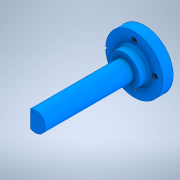
# Autodesk Inventor part: BM-AX12
Saved by Autodesk Inventor 2021 (Build 250183000, 183)
## iProperties
Created: 2021-10-29
Part Number: BM-AX12
Material: PETG
Document SubType Name: Modeling
Designer: Alcatraz
Density: 1.27 g/cm^3
Appearance: Genérico
Author: Alcatraz
Autodesk Inventor part; units mm, degrees
ref_plane "XZ Plane" through (0, 0, 0) normal (0, 1, 0) x (-1, 0, 0)
ref_plane "XY Plane" through (0, 0, 0) normal (0, 0, 1) x (1, 0, 0)
sketch "Boceto1" plane through (0, 0, 0) normal (0, 0, 1) x (1, 0, 0)
  circle A0 centre (0, 0) radius 11
  dimension "DIAMETROBRIDA" = 22
  constraints: 1 centre point, 1 coincident
  measures "DIAMETROBRIDA" diameter of A0
extrude "Extrusión1" add sketch "Boceto1" along normal blind 4
sketch "Boceto2" plane through (0, 0, 4) normal (0, 0, 1) x (1, 0, 0)
  circle A0 centre (0, 8) radius 1.05
  circle A1 centre (-8, 0) radius 1.05
  circle A2 centre (8, 0) radius 1.05
  circle A3 centre (0, -8) radius 1.05
  circle A4 centre (0, 0) radius 11 projected
  dimension "d7" = 2.1
  dimension "d8" = 2.1
  dimension "d9" = 2.1
  dimension "d10" = 2.1
  dimension "DistanciaBarrenos" = 8
  dimension "d31" = 8
  dimension "d32" = 8
  dimension "d33" = 8
  constraints: 4 centre point
  measures "d7" diameter of A0
  measures "d8" diameter of A1
  measures "d9" diameter of A2
  measures "d10" diameter of A3
  measures "DistanciaBarrenos" distance of A1.centre A4.centre
  measures "d31" distance of point (0, 0) A0.centre
  measures "d32" distance of A2.centre point (0, 0)
  measures "d33" distance of A3.centre point (0, 0)
hole "Agujero1" at (0, 8, 4) at (-8, 0, 4) at (8, 0, 4) at (0, -8, 4) direction (0, 0, -1) diameter 2.013 end through all thread size "M2.5x0.45" class "6H" standard "ISO Metric profile"
sketch "Boceto3" plane through (0, 0, 4) normal (0, 0, 1) x (1, 0, 0)
  circle A0 centre (0, 0) radius 6
  dimension "DIAMETROBASE" = 12
  constraints: 1 centre point, 1 coincident
  measures "DIAMETROBASE" diameter of A0
extrude "Extrusión2" add sketch "Boceto3" along normal blind 4
sketch "Boceto4" plane through (0, 0, 8) normal (0, 0, 1) x (1, 0, 0)
  arc A0 (-1.9, -3.2909) -> (-1.9, 3.2909) centre (0, 0) ccw
  line L0 (0, 0) -> (-2, 0)
  line L1 (-1.9, 3.2909) -> (-1.9, -3.2909)
  circle A1 centre (0, 0) radius 6 projected
  dimension "DIAMETROEJE" = 7.6
  dimension "d29" = 1.9
  dimension "d38" = 2
  constraints: 4 end point, 2 point on circle, 1 centre point, 1 coincident, 1 concentric, 1 horizontal, 1 vertical
  measures "DIAMETROEJE" diameter of A0
  measures "d29" distance from line of L0.start L1
  measures "d38" distance of L0.start L0.end
extrude "Extrusión3" add sketch "Boceto4" along normal blind 34 contours L1 A0
ref_plane "Plano de trabajo1" through (-11, 0, 0) normal (1, 0, 0) x (0, 1, 0)
sketch "Boceto7" plane through (-11, 0, 0) normal (1, 0, 0) x (0, 1, 0)
  line L0 (0.5, 4) -> (-0.5, 4)
  line L1 (-0.5, 4) -> (-0.5, 0)
  line L2 (-0.5, 0) -> (0.5, 0)
  line L3 (0.5, 0) -> (0.5, 4)
  line L4 (0.5, 4) -> (-0.5, 0) construction
  line L5 (-0.5, 4) -> (0.5, 0) construction
  point P0 (0, 0)
  point P1 (0, 2)
  dimension "d34" = 1
  dimension "d35" = 4
  constraints: 12 end point, 2 midpoint, 2 parallel, 1 horizontal, 1 perpendicular
  measures "d34" distance of L2.end L1.end
  measures "d35" distance of L1.end L0.end
extrude "Extrusión4" cut sketch "Boceto7" along normal blind 0.5
fillet "Empalme5" radius 1 2 edges at (-1.9, 0, 8) (-6, 0, 4)
equation "\"d8\" = d7"
equation "\"d9\" = d7"
equation "\"d10\" = d7"
equation "\"d31\" = DistanciaBarrenos"
equation "\"d32\" = DistanciaBarrenos"
equation "\"d33\" = DistanciaBarrenos"
equation "\"d29\" = 0.25 * DIAMETROEJE"
